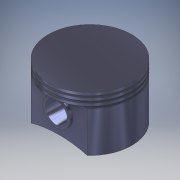
# Autodesk Inventor part: Part12
Saved by Autodesk Inventor 2019 (Build 230136000, 136)
## iProperties
Created: 2022-01-28
Part Number: Part12
Material: Generic
Document SubType Name: Modeling
Designer: Sepehr
Density: 1 g/cm^3
Appearance: Default
Author: Sepehr
Autodesk Inventor part; units mm, degrees
ref_plane "YZ Plane" through (0, 0, 0) normal (1, 0, 0) x (0, 1, 0)
ref_plane "XZ Plane" through (0, 0, 0) normal (0, 1, 0) x (-1, 0, 0)
ref_plane "XY Plane" through (0, 0, 0) normal (0, 0, 1) x (1, 0, 0)
sketch "Sketch1" plane through (0, 0, 0) normal (0, 1, 0) x (-1, 0, 0)
  line L0 (0, -1700) -> (1549.1933, -1700)
  line L1 (1549.1933, -1700) -> (-1549.1933, -1700)
  line L2 (0, 1700) -> (1549.1933, 1700)
  line L3 (0, 1700) -> (-1549.1933, 1700)
  arc A0 (-1549.1933, 1700) -> (-1549.1933, -1700) centre (0, 0) ccw
  arc A1 (1549.1933, -1700) -> (1549.1933, 1700) centre (0, 0) ccw
  line L4 (0, 785.9327) -> (774.5967, 785.9327)
  line L5 (774.5967, 785.9327) -> (774.5967, 1342.5722)
  line L6 (774.5967, 1342.5722) -> (1549.1933, 1342.5722)
  line L7 (0, 785.9327) -> (-774.597, 785.9327)
  line L8 (-774.597, 785.9327) -> (-774.597, 1342.5722)
  line L9 (-774.597, 1342.5722) -> (-1549.1933, 1342.5722)
  line L10 (-1549.1933, -1342.5722) -> (-774.597, -1342.5722)
  line L11 (1549.1933, -1342.5722) -> (774.5967, -1342.5722)
  line L12 (774.5967, -1342.5722) -> (774.5967, -785.9332)
  line L13 (774.5967, -785.9332) -> (-774.597, -785.9332)
  line L14 (-774.597, -785.9332) -> (-774.597, -1342.5722)
  arc A2 (-1549.1933, 1342.5722) -> (-1549.1933, -1342.5722) centre (0, 0) ccw
  arc A3 (1549.1933, -1342.5722) -> (1549.1933, 1342.5722) centre (0, 0) ccw
  constraints: 30 end point, 8 point on circle, 5 perpendicular, 4 centre point, 2 horizontal, 2 vertical, 1 coincident, 1 point on line
extrude "Extrusion1" add sketch "Sketch1" along normal blind 2250
sketch "Sketch2" plane through (0, 2250, 0) normal (0, 1, 0) x (1, 0, 0)
  circle A0 centre (0, 0) radius 2125
  dimension "d8" = 4250
  constraints: 1 centre point, 1 coincident
  measures "d8" diameter of A0
extrude "Extrusion2" add sketch "Sketch2" along normal blind 100
sketch "Sketch3" plane through (0, 2350, 0) normal (0, 1, 0) x (1, 0, 0)
  circle A0 centre (0, 0) radius 2300
  dimension "d11" = 4600
  constraints: 1 centre point, 1 coincident
  measures "d11" diameter of A0
extrude "Extrusion3" add sketch "Sketch3" along normal blind 150
sketch "Sketch4" plane through (0, 2500, 0) normal (0, 1, 0) x (1, 0, 0)
  circle A0 centre (0, 0) radius 2125
  dimension "d14" = 4250
  constraints: 1 centre point, 1 coincident
  measures "d14" diameter of A0
extrude "Extrusion4" add sketch "Sketch4" along normal blind 100
sketch "Sketch5" plane through (0, 2600, 0) normal (0, 1, 0) x (1, 0, 0)
  circle A0 centre (0, 0) radius 2300
  dimension "d17" = 4600
  constraints: 1 centre point, 1 coincident
  measures "d17" diameter of A0
extrude "Extrusion5" add sketch "Sketch5" along normal blind 150
sketch "Sketch6" plane through (0, 2750, 0) normal (0, 1, 0) x (1, 0, 0)
  circle A0 centre (0, 0) radius 2125
  dimension "d20" = 4250
  constraints: 1 centre point, 1 coincident
  measures "d20" diameter of A0
extrude "Extrusion6" add sketch "Sketch6" along normal blind 100
sketch "Sketch7" plane through (0, 2850, 0) normal (0, 1, 0) x (1, 0, 0)
  circle A0 centre (0, 0) radius 2300
  dimension "d23" = 4600
  constraints: 1 centre point, 1 coincident
  measures "d23" diameter of A0
extrude "Extrusion7" add sketch "Sketch7" along normal blind 150
sketch "Sketch8" plane through (-1549.1933, 0, 1700) normal (0, 0, 1) x (1, 0, 0)
  line L0 (3098.3867, 0) -> (0, 0) projected
  arc A0 (3098.3867, 0) -> (0, 0) centre (1549.1933, -5589.2754) ccw
  line L1 (0, 0) -> (3098.3867, 0)
  point P0 (1549.1933, 0)
  dimension "d26" = 5800
  constraints: 2 end point, 2 point on circle, 1 centre point, 1 horizontal
  measures "d26" radius of A0
extrude "Extrusion8" cut sketch "Sketch8" against normal blind 10000
sketch "Sketch9" plane through (-1275, 2250, 1700) normal (0, 0, 1) x (1, 0, 0)
  line L0 (1275, -2250) -> (1275, -900)
  circle A0 centre (1275, -900) radius 600
  dimension "d29" = 1350
  dimension "d30" = 1200
  constraints: 2 end point, 1 centre point, 1 coincident, 1 vertical
  measures "d29" distance of L0.start L0.end
  measures "d30" diameter of A0
extrude "Extrusion9" cut sketch "Sketch9" against normal blind 10000
sketch "Sketch10" plane through (-1275, 2250, 1700) normal (0, 0, 1) x (1, 0, 0)
  circle A0 centre (1275, -900) radius 600 projected
  circle A1 centre (1275, -900) radius 600
  circle A2 centre (1275, -900) radius 750
  point P0 (1275, -2250)
  dimension "d33" = 1200
  dimension "d34" = 1500
  constraints: 2 centre point, 2 coincident
  measures "d33" diameter of A1
  measures "d34" diameter of A2
extrude "Extrusion10" add sketch "Sketch10" along normal blind 150
body "Solid1"
